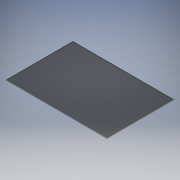
# Autodesk Inventor part: Black Glass Piece
Saved by Autodesk Inventor 2016 (Build 200138000, 138)
## iProperties
Created: 2015-11-19
Part Number: Black Glass Piece
Material: 玻璃
Document SubType Name: Modeling
Designer: Shawn Shi Feng
Density: 2.18 g/cm^3
Appearance: 清晰
Author: Shawn Shi Feng
Autodesk Inventor part; units mm, degrees
ref_plane "YZ Plane" through (0, 0, 0) normal (1, 0, 0) x (0, 1, 0)
ref_plane "XZ Plane" through (0, 0, 0) normal (0, 1, 0) x (-1, 0, 0)
ref_plane "XY Plane" through (0, 0, 0) normal (0, 0, 1) x (1, 0, 0)
sketch "草图1" plane through (0, 0, 0) normal (0, 0, 1) x (1, 0, 0)
  line L0 (-374.5736, 202.2432) -> (380.4264, 202.2432)
  line L1 (380.4264, 202.2432) -> (380.4264, -297.7568)
  line L2 (380.4264, -297.7568) -> (-374.5736, -297.7568)
  line L3 (-374.5736, -297.7568) -> (-374.5736, 202.2432)
  point P0 (0, 0)
  dimension "d0" = 755
  dimension "d1" = 500
  constraints: 8 end point, 2 parallel, 1 horizontal, 1 perpendicular
  measures "d0" distance of L1.end L2.end
  measures "d1" distance of L0.end L1.end
extrude "拉伸1" add sketch "草图1" along normal blind 5
